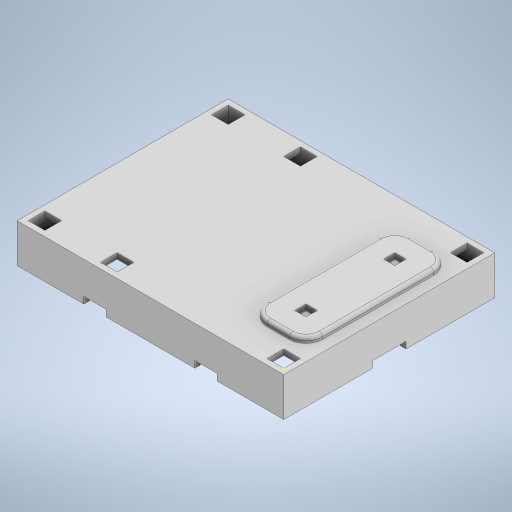
# Autodesk Inventor part: bovenkant
Saved by Autodesk Inventor 2023 (Build 270158000, 158)
## iProperties
Created: 2023-06-01
Part Number: bovenkant
Material: Generic
Document SubType Name: Modeling
Designer: Prestige
Density: 1 g/cm^3
Appearance: Default
Author: Prestige
Autodesk Inventor part; units mm, degrees
ref_plane "YZ Plane" through (0, 0, 0) normal (1, 0, 0) x (0, 1, 0)
ref_plane "XZ Plane" through (0, 0, 0) normal (0, 1, 0) x (-1, 0, 0)
ref_plane "XY Plane" through (0, 0, 0) normal (0, 0, 1) x (1, 0, 0)
sketch "Sketch1" plane through (0, 0, 0) normal (0, 1, 0) x (-1, 0, 0)
  line L0 (0, 0) -> (230, 0)
  line L1 (230, 0) -> (230, -180)
  line L2 (230, -180) -> (0, -180)
  line L3 (0, -180) -> (0, 0)
  line L4 (235, -185) -> (-5, -185)
  line L5 (-5, -185) -> (-5, 5)
  line L6 (-5, 5) -> (235, 5)
  line L7 (235, 5) -> (235, -185)
  line L8 (235, -75) -> (230, -75)
  line L9 (230, -75) -> (230, -105)
  line L10 (230, -105) -> (235, -105)
  line L11 (235, -105) -> (235, -75)
  line L12 (175, -180) -> (155, -180)
  line L13 (155, -180) -> (155, -185)
  line L14 (155, -185) -> (175, -185)
  line L15 (175, -185) -> (175, -180)
  line L16 (115, -180) -> (95, -180)
  line L17 (95, -185) -> (115, -185)
  line L18 (-5, -73.4747) -> (0, -73.4747)
  line L19 (0, -73.4747) -> (0, -111.2886)
  line L20 (0, -111.2886) -> (-5, -111.2886)
  line L21 (-5, -111.2886) -> (-5, -73.4747)
  line L22 (175, 0) -> (155, 0)
  line L23 (155, 0) -> (155, 5)
  line L24 (155, 5) -> (175, 5)
  line L25 (175, 5) -> (175, 0)
  line L26 (75, 0) -> (55, 0)
  line L27 (55, 0) -> (55, 5)
  line L28 (55, 5) -> (75, 5)
  line L29 (75, 5) -> (75, 0)
  line L30 (75, -180) -> (55, -180)
  line L31 (55, -180) -> (55, -185)
  line L32 (55, -185) -> (75, -185)
  line L33 (75, -185) -> (75, -180)
  point P0 (232.5, -75)
  point P1 (232.5, -105)
  point P2 (175, 2.5)
  point P3 (155, 2.5)
  point P4 (55, 2.5)
  point P5 (75, 2.5)
  point P6 (155, -182.5)
  point P7 (175, -182.5)
  point P8 (55, -182.5)
  point P9 (75, -182.5)
  point P10 (-5, -111.2886)
  point P11 (0, -73.4747)
  dimension "d0" = 180
  dimension "d1" = 230
  dimension "d2" = 5
  dimension "d3" = 5
  dimension "d4" = 5
  dimension "d5" = 5
  dimension "d6" = 30
  dimension "d7" = 75
  dimension "d8" = 75
  dimension "d9" = 20
  dimension "d10" = 20
  dimension "d12" = 20
  dimension "d14" = 80
  dimension "d15" = 55
  dimension "d16" = 55
  dimension "d17" = 20
  dimension "d18" = 80
  constraints: 68 end point, 17 parallel, 13 point on line, 11 midpoint, 9 horizontal, 8 perpendicular
  measures "d0" distance of L2.end L0.start
  measures "d1" distance of L0.start L0.end
  measures "d2" distance between parallel lines of L1 L7
  measures "d3" distance between parallel lines of L2 L4
  measures "d4" distance between parallel lines of L3 L5
  measures "d5" distance between parallel lines of L0 L6
  measures "d6" distance from line of point (232.5, -75) L10
  measures "d7" distance between parallel lines of L0 L8
  measures "d8" distance from line of L2 point (232.5, -105)
  measures "d9" distance of point (175, 2.5) point (155, 2.5)
  measures "d10" distance of point (55, 2.5) point (75, 2.5)
  measures "d12" distance of point (155, -182.5) point (175, -182.5)
  measures "d14" distance between parallel lines of L23 L29
  measures "d15" distance between parallel lines of L1 L25
  measures "d16" distance between parallel lines of L1 L15
  measures "d17" distance of point (55, -182.5) point (75, -182.5)
  measures "d18" distance from line of point (155, -182.5) L33
extrude "Extrusion1" add sketch "Sketch1" along normal blind 6 contours L3 L18 L5 L6 L27 L0 | L29 L6 L23 L0 | L3 L2 L31 L4 L5 L20 | L25 L6 L7 L8 L1 L0 | L2 L13 L4 L33 | L10 L7 L4 L15 L2 L1
sketch "Sketch2" plane through (0, 6, 0) normal (0, 1, 0) x (1, 0, 0)
  line L0 (0, 180) -> (0, 111.2886) projected
  line L1 (-175, 0) -> (-230, 0) projected
  line L2 (0, 180) -> (-230, 180)
  line L3 (-230, 180) -> (-230, 0)
  line L4 (-230, 0) -> (0, 0)
  line L5 (0, 0) -> (0, 180)
  line L6 (-235, 75) -> (-235, -5) projected
  line L7 (5, 111.2886) -> (5, 185) projected
  line L8 (-235, -5) -> (5, -5)
  line L9 (5, -5) -> (5, 185)
  line L10 (5, 185) -> (-235, 185)
  line L11 (-235, 185) -> (-235, -5)
  point P0 (0, 0)
  constraints: 16 end point, 4 parallel, 2 horizontal, 2 perpendicular
extrude "Extrusion2" add sketch "Sketch2" along normal blind 24
sketch "Sketch3" plane through (0, 30, 0) normal (0, 1, 0) x (1, 0, 0)
  line L0 (-235, -5) -> (5, -5) projected
  line L1 (5, 185) -> (-235, 185) projected
  line L2 (-235, -5) -> (5, -5)
  line L3 (5, -5) -> (5, 185)
  line L4 (5, 185) -> (-235, 185)
  line L5 (-235, 185) -> (-235, -5)
  point P0 (0, 0)
  constraints: 8 end point, 2 parallel, 1 horizontal, 1 perpendicular
extrude "Extrusion3" add sketch "Sketch3" along normal blind 5
sketch "Sketch4" plane through (0, 35, 0) normal (0, 1, 0) x (1, 0, 0)
  line L0 (-5, 25) -> (-55, 25)
  line L1 (-55, 25) -> (-55, 155)
  line L2 (-55, 155) -> (-5, 155)
  line L3 (-5, 155) -> (-5, 25)
  line L4 (5, 185) -> (-235, 185) projected
  line L5 (-235, -5) -> (5, -5) projected
  line L6 (5, -5) -> (5, 185) projected
  point P0 (0, 0)
  dimension "d25" = 130
  dimension "d26" = 30
  dimension "d27" = 30
  dimension "d28" = 10
  dimension "d29" = 50
  constraints: 8 end point, 2 parallel, 1 horizontal, 1 perpendicular
  measures "d25" distance of L0.end L1.end
  measures "d26" distance between parallel lines of L4 L2
  measures "d27" distance between parallel lines of L5 L0
  measures "d28" distance between parallel lines of L6 L3
  measures "d29" distance of L1.end L2.end
extrude "Extrusion4" add sketch "Sketch4" along normal blind 5
fillet "Fillet1" radius 15 4 edges at (-5, 37.5, -25) (-55, 37.5, -25) (-5, 37.5, -155) (-55, 37.5, -155)
fillet "Fillet2" radius 3 8 edges at (-9.3934, 40, -150.6066) (-30, 40, -155) (-50.6066, 40, -150.6066) (-55, 40, -90) (-50.6066, 40, -29.3934) (-30, 40, -25) (-9.3934, 40, -29.3934) (-5, 40, -90)
sketch "Sketch5" plane through (0, 40, 0) normal (0, 1, 0) x (1, 0, 0)
  line L0 (-25, 125) -> (-35, 125)
  line L1 (-35, 125) -> (-35, 135)
  line L2 (-35, 135) -> (-25, 135)
  line L3 (-25, 135) -> (-25, 125)
  line L4 (-20, 155) -> (-40, 155) projected
  line L5 (-55, 140) -> (-55, 40) projected
  line L6 (-35, 45) -> (-25, 45)
  line L7 (-25, 45) -> (-25, 55)
  line L8 (-25, 55) -> (-35, 55)
  line L9 (-35, 55) -> (-35, 45)
  line L10 (-40, 25) -> (-20, 25) projected
  point P0 (0, 0)
  point P1 (-30, 125)
  point P2 (-30, 155)
  point P3 (-30, 135)
  point P4 (-30, 45)
  point P5 (-35, 50)
  point P6 (-30, 25)
  dimension "d34" = 10
  dimension "d35" = 10
  dimension "d36" = 20
  dimension "d37" = 20
  dimension "d40" = 10
  dimension "d41" = 10
  dimension "d42" = 20
  dimension "d43" = 20
  constraints: 16 end point, 6 midpoint, 4 parallel, 2 horizontal, 2 perpendicular
  measures "d34" distance between parallel lines of L3 L1
  measures "d35" distance from line of point (-30, 125) L2
  measures "d36" distance of point (-30, 155) point (-30, 135)
  measures "d37" distance between parallel lines of L5 L1
  measures "d40" distance between parallel lines of L7 L9
  measures "d41" distance from line of point (-30, 45) L8
  measures "d42" distance from line of L5 point (-35, 50)
  measures "d43" distance of point (-30, 25) point (-30, 45)
extrude "Extrusion5" cut sketch "Sketch5" against normal blind 5
sketch "Sketch6" plane through (0, 35, 0) normal (0, 1, 0) x (1, 0, 0)
  line L0 (0, 0) -> (-55, 0) projected
  line L1 (0, 0) -> (-15, 0)
  line L2 (-15, 0) -> (-15, 15)
  line L3 (-15, 15) -> (0, 15)
  line L4 (0, 15) -> (0, 0)
  line L5 (5, -5) -> (5, 185) projected
  line L6 (0, 0) -> (-230, 0) projected
  line L7 (-230, 0) -> (-215, 0)
  line L8 (-215, 0) -> (-215, 15)
  line L9 (-215, 15) -> (-230, 15)
  line L10 (-230, 15) -> (-230, 0)
  line L11 (-230, 180) -> (-215, 180)
  line L12 (-215, 180) -> (-215, 165)
  line L13 (-215, 165) -> (-230, 165)
  line L14 (-230, 165) -> (-230, 180)
  line L15 (-165, 0) -> (-150, 0)
  line L16 (-150, 0) -> (-150, 15)
  line L17 (-150, 15) -> (-165, 15)
  line L18 (-165, 15) -> (-165, 0)
  line L19 (-165, 180) -> (-150, 180)
  line L20 (-150, 180) -> (-150, 165)
  line L21 (-150, 165) -> (-165, 165)
  line L22 (-165, 165) -> (-165, 180)
  line L23 (0, 180) -> (-15, 180)
  line L24 (-15, 180) -> (-15, 165)
  line L25 (-15, 165) -> (0, 165)
  line L26 (0, 165) -> (0, 180)
  point P0 (-222.5, 0)
  point P1 (-222.5, 15)
  dimension "d46" = 15
  dimension "d47" = 15
  dimension "d51" = 15
  dimension "d52" = 15
  dimension "d53" = 15
  dimension "d54" = 15
  dimension "d55" = 15
  dimension "d56" = 15
  dimension "d57" = 15
  dimension "d58" = 15
  dimension "d59" = 50
  dimension "d64" = 15
  dimension "d65" = 15
  constraints: 48 end point, 12 parallel, 6 horizontal, 6 perpendicular, 2 midpoint, 2 point on line
  measures "d46" distance of L1.end L2.end
  measures "d47" distance of L2.end L3.end
  measures "d51" distance of point (-222.5, 0) point (-222.5, 15)
  measures "d52" distance of L8.end L9.end
  measures "d53" distance of L11.end L12.end
  measures "d54" distance of L12.end L13.end
  measures "d55" distance of L17.end L15.start
  measures "d56" distance of L16.end L17.end
  measures "d57" distance of L20.end L21.end
  measures "d58" distance of L19.end L20.end
  measures "d59" distance between parallel lines of L12 L22
  measures "d64" distance of L24.end L25.end
  measures "d65" distance of L23.end L24.end
extrude "Extrusion6" cut sketch "Sketch6" against normal blind 5
sketch "Sketch7" plane through (5, 0, 5) normal (1, 0, 0) x (0, 0, -1)
  line L0 (110, 0) -> (110, 6) projected
  line L1 (110, 0) -> (120.7181, 0)
  line L2 (120.7181, 0) -> (120.7181, 6)
  line L3 (120.7181, 6) -> (110, 6)
  line L4 (110, 6) -> (110, 0)
  line L5 (80, 0) -> (80, 6) projected
  line L6 (80, 0) -> (68.1544, 0)
  line L7 (68.1544, 0) -> (68.1544, 6)
  line L8 (68.1544, 6) -> (80, 6)
  line L9 (80, 6) -> (80, 0)
  point P0 (5, 0)
  constraints: 16 end point, 4 parallel, 2 horizontal, 2 perpendicular
extrude "Extrusion7" add sketch "Sketch7" against normal blind 5
sketch "Sketch8" plane through (0, 35, 0) normal (0, 1, 0) x (1, 0, 0)
  point P0 (0, 0)
body "Solid1"
